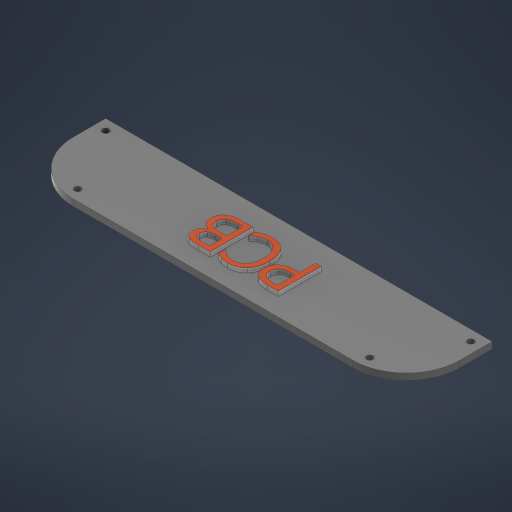
# Autodesk Inventor part: pcb
Saved by Autodesk Inventor 2024 (Build 280153000, 153)
## iProperties
Created: 2023-07-13
Part Number: pcb
Material: 일반
Document SubType Name: Modeling
Designer: 6gioc
Density: 1 g/cm^3
Appearance: 기본값
Author: 6gioc
Autodesk Inventor part; units mm, degrees
ref_plane "YZ Plane" through (0, 0, 0) normal (1, 0, 0) x (0, 1, 0)
ref_plane "XZ Plane" through (0, 0, 0) normal (0, 1, 0) x (-1, 0, 0)
ref_plane "XY Plane" through (0, 0, 0) normal (0, 0, 1) x (1, 0, 0)
sketch "스케치1" plane through (0, 0, 0) normal (0, 1, 0) x (-1, 0, 0)
  line L0 (-25, 0) -> (-155, 0)
  line L1 (-180, -25) -> (-180, -40)
  line L2 (-180, -40) -> (0, -40)
  line L3 (0, -40) -> (0, -25)
  arc A0 (0, -25) -> (-25, 0) centre (-25, -25) ccw
  arc A1 (-155, 0) -> (-180, -25) centre (-155, -25) ccw
  circle A2 centre (-5, -35) radius 1.5
  circle A3 centre (-5, -35) radius 2.5
  circle A4 centre (-5, -22) radius 1.5
  circle A5 centre (-5, -22) radius 2.5
  circle A6 centre (-22, -5) radius 1.5
  circle A7 centre (-22, -5) radius 2.5
  line L4 (-90, -40) -> (-90, 0)
  circle A8 centre (-90, -35) radius 2.5
  circle A9 centre (-90, -5) radius 2.5
  circle A10 centre (-47.5, -35) radius 2.5
  circle A11 centre (-175, -35) radius 1.5
  circle A12 centre (-175, -35) radius 2.5
  circle A13 centre (-175, -22) radius 1.5
  circle A14 centre (-175, -22) radius 2.5
  circle A15 centre (-158, -5) radius 1.5
  circle A16 centre (-158, -5) radius 2.5
  circle A17 centre (-132.5, -35) radius 2.5
  point P0 (0, 0)
  point P1 (-180, 0)
  dimension "d0" = 180
  dimension "d1" = 40
  dimension "d2" = 25
  dimension "d3" = 3
  dimension "d4" = 5
  dimension "d5" = 3
  dimension "d6" = 5
  dimension "d7" = 3
  dimension "d8" = 5
  dimension "d9" = 5
  dimension "d10" = 5
  dimension "d11" = 5
  dimension "d12" = 5
  dimension "d13" = 5
  dimension "d14" = 5
  dimension "d15" = 5
  dimension "d16" = 5
  dimension "d17" = 5
  dimension "d18" = 85
  dimension "d19" = 42.5
  dimension "d20" = 3
  dimension "d21" = 3
  constraints: 18 centre point, 10 end point, 7 symmetric about line, 6 coincident, 6 point on line, 4 point on circle, 4 tangent, 2 midpoint, 2 parallel, 1 equal radius, 1 horizontal, 1 horizontal alignment, 1 perpendicular, 7 other
  measures "d0" distance of L2.end L1.end
  measures "d1" distance of L1.end point (-180, 0)
  measures "d2" radius of A0
  measures "d3" diameter of A2
  measures "d4" diameter of A3
  measures "d5" diameter of A4
  measures "d6" diameter of A5
  measures "d7" diameter of A6
  measures "d8" diameter of A7
  measures "d9" diameter of A8
  measures "d10" diameter of A9
  measures "d11" diameter of A10
  measures "d12" distance from line of L2 A3.centre
  measures "d13" distance from line of A3.centre L3
  measures "d14" distance from line of L3 A5.centre
  measures "d15" distance from line of L0 A7.centre
  measures "d16" distance from line of L2 A8.centre
  measures "d17" distance from line of L0 A9.centre
  measures "d18" distance of A8.centre A2.centre
  measures "d19" distance of A8.centre A10.centre
  measures "d20" horizontal distance of L0.start A7.centre
  measures "d21" vertical distance of L3.end A5.centre
extrude "돌출1" add sketch "스케치1" along normal blind 3 contours A0 L3 L2 L4 A8 A9 L0 | L4 A9 A8 L2 L1 A1 L0 | A9 L4 | L4 A9 | A8 L4 | L4 A8 | A3 | A4 | A5 | A7 | A10 | A12 | A13 | A14 | A16 | A17
sketch "스케치2" plane through (0, 3, 0) normal (0, 1, 0) x (1, 0, 0)
  line L0 (113.9465, 8.0671) -> (66.0535, 8.0671) construction
  line L1 (66.0535, 8.0671) -> (66.0535, 31.9329) construction
  line L2 (66.0535, 31.9329) -> (113.9465, 31.9329) construction
  line L3 (113.9465, 31.9329) -> (113.9465, 8.0671) construction
  line L4 (0, 40) -> (0, 25) projected
  line L5 (180, 40) -> (0, 40) projected
  spline S0 degree 2 poles (99.2788, 14.4529) (99.2788, 15.7494) (100.2026, 18.0833) (101.0292, 18.8937) knots 0 0 0 1 2 2 2
  spline S1 degree 2 poles (101.0292, 18.8937) (102.0664, 19.9148) (104.8703, 20.9682) (107.0097, 20.9682) knots 0 0 0 1 2 2 2
  line L6 (107.0097, 20.9682) -> (109.2626, 20.9682)
  line L7 (109.2626, 20.9682) -> (109.2626, 28.4237)
  line L8 (109.2626, 28.4237) -> (111.9206, 28.4237)
  line L9 (111.9206, 28.4237) -> (111.9206, 8.4237)
  line L10 (111.9206, 8.4237) -> (106.8963, 8.4237)
  spline S2 degree 2 poles (106.8963, 8.4237) (105.1135, 8.4237) (102.6175, 9.0071) (101.6613, 9.6717) knots 0 0 0 1 2 2 2
  spline S3 degree 2 poles (101.6613, 9.6717) (100.5429, 10.4334) (99.2788, 12.7835) (99.2788, 14.4529) knots 0 0 0 1 2 2 2
  spline S4 degree 2 poles (102.0502, 14.5339) (102.0502, 13.4966) (102.7634, 11.9731) (103.4927, 11.4869) knots 0 0 0 1 2 2 2
  spline S5 degree 2 poles (103.4927, 11.4869) (104.1248, 11.0655) (105.8104, 10.7251) (107.0583, 10.7251) knots 0 0 0 1 2 2 2
  line L11 (107.0583, 10.7251) -> (109.2626, 10.7251)
  line L12 (109.2626, 10.7251) -> (109.2626, 18.6992)
  line L13 (109.2626, 18.6992) -> (107.4473, 18.6992)
  spline S6 degree 2 poles (107.4473, 18.6992) (105.8266, 18.6992) (103.8331, 18.1806) (103.1848, 17.4999) knots 0 0 0 1 2 2 2
  spline S7 degree 2 poles (103.1848, 17.4999) (102.5851, 16.9002) (102.0502, 15.4901) (102.0502, 14.5339) knots 0 0 0 1 2 2 2
  spline S8 degree 2 poles (88.9384, 28.7802) (90.8833, 28.7802) (94.1734, 27.4674) (95.3728, 26.1546) knots 0 0 0 1 2 2 2
  spline S9 degree 2 poles (95.3728, 26.1546) (96.5721, 24.858) (97.8849, 20.9682) (97.8849, 18.4399) knots 0 0 0 1 2 2 2
  spline S10 degree 2 poles (97.8849, 18.4399) (97.8849, 15.9277) (96.6045, 12.2) (95.389, 10.8224) knots 0 0 0 1 2 2 2
  spline S11 degree 2 poles (95.389, 10.8224) (94.1896, 9.4772) (90.9157, 8.0671) (88.8898, 8.0671) knots 0 0 0 1 2 2 2
  spline S12 degree 2 poles (88.8898, 8.0671) (87.8849, 8.0671) (86.1183, 8.3588) (85.3728, 8.5858) knots 0 0 0 1 2 2 2
  spline S13 degree 2 poles (85.3728, 8.5858) (84.7245, 8.7964) (83.3793, 9.3961) (82.7147, 9.7527) knots 0 0 0 1 2 2 2
  line L14 (82.7147, 9.7527) -> (82.7147, 12.9618)
  line L15 (82.7147, 12.9618) -> (82.9254, 12.9618)
  spline S14 degree 2 poles (82.9254, 12.9618) (83.282, 12.6376) (84.3841, 11.73) (85.1783, 11.2924) knots 0 0 0 1 2 2 2
  spline S15 degree 2 poles (85.1783, 11.2924) (85.94, 10.871) (87.7391, 10.3362) (88.906, 10.3362) knots 0 0 0 1 2 2 2
  spline S16 degree 2 poles (88.906, 10.3362) (90.1864, 10.3362) (92.4716, 11.3896) (93.3306, 12.3945) knots 0 0 0 1 2 2 2
  spline S17 degree 2 poles (93.3306, 12.3945) (94.1734, 13.4156) (95.1135, 16.5112) (95.1135, 18.4399) knots 0 0 0 1 2 2 2
  spline S18 degree 2 poles (95.1135, 18.4399) (95.1135, 20.4982) (94.1248, 23.4642) (93.2658, 24.4853) knots 0 0 0 1 2 2 2
  spline S19 degree 2 poles (93.2658, 24.4853) (92.423, 25.4739) (90.1702, 26.4788) (88.906, 26.4788) knots 0 0 0 1 2 2 2
  spline S20 degree 2 poles (88.906, 26.4788) (87.7553, 26.4788) (85.7942, 25.9115) (85.0324, 25.4901) knots 0 0 0 1 2 2 2
  spline S21 degree 2 poles (85.0324, 25.4901) (84.3031, 25.0687) (83.2172, 24.1935) (82.9092, 23.8856) knots 0 0 0 1 2 2 2
  line L16 (82.9092, 23.8856) -> (82.7147, 23.8856)
  line L17 (82.7147, 23.8856) -> (82.7147, 27.0623)
  spline S22 degree 2 poles (82.7147, 27.0623) (83.3793, 27.3702) (84.5462, 27.9375) (85.3728, 28.1968) knots 0 0 0 1 2 2 2
  spline S23 degree 2 poles (85.3728, 28.1968) (86.248, 28.4885) (87.7391, 28.7802) (88.9384, 28.7802) knots 0 0 0 1 2 2 2
  spline S24 degree 2 poles (66.6694, 22.2811) (66.6694, 23.7721) (67.8039, 26.0574) (68.7439, 26.8029) knots 0 0 0 1 2 2 2
  spline S25 degree 2 poles (68.7439, 26.8029) (69.8784, 27.6781) (72.4554, 28.4237) (74.4976, 28.4237) knots 0 0 0 1 2 2 2
  line L18 (74.4976, 28.4237) -> (80.235, 28.4237)
  line L19 (80.235, 28.4237) -> (80.235, 8.4237)
  line L20 (80.235, 8.4237) -> (74.9352, 8.4237)
  spline S26 degree 2 poles (74.9352, 8.4237) (72.7958, 8.4237) (70.6564, 8.6992) (69.684, 9.234) knots 0 0 0 1 2 2 2
  spline S27 degree 2 poles (69.684, 9.234) (68.5981, 9.8013) (67.6094, 11.6652) (67.6094, 12.9293) knots 0 0 0 1 2 2 2
  spline S28 degree 2 poles (67.6094, 12.9293) (67.6094, 14.3394) (69.1005, 16.576) (70.4133, 17.2081) knots 0 0 0 1 2 2 2
  line L21 (70.4133, 17.2081) -> (70.4133, 17.3054)
  spline S29 degree 2 poles (70.4133, 17.3054) (68.6305, 17.7916) (66.6694, 20.3686) (66.6694, 22.2811) knots 0 0 0 1 2 2 2
  spline S30 degree 2 poles (69.4408, 22.3945) (69.4408, 21.26) (70.0891, 19.8013) (71.0616, 19.2827) knots 0 0 0 1 2 2 2
  spline S31 degree 2 poles (71.0616, 19.2827) (71.6937, 18.9585) (73.1848, 18.764) (74.5624, 18.764) knots 0 0 0 1 2 2 2
  line L22 (74.5624, 18.764) -> (77.577, 18.764)
  line L23 (77.577, 18.764) -> (77.577, 26.1546)
  line L24 (77.577, 26.1546) -> (75.4214, 26.1546)
  spline S32 degree 2 poles (75.4214, 26.1546) (73.671, 26.1546) (71.6613, 25.8305) (70.8833, 25.3118) knots 0 0 0 1 2 2 2
  spline S33 degree 2 poles (70.8833, 25.3118) (70.1378, 24.777) (69.4408, 23.448) (69.4408, 22.3945) knots 0 0 0 1 2 2 2
  spline S34 degree 2 poles (70.3809, 13.3021) (70.3809, 12.589) (70.8671, 11.5193) (71.4019, 11.2114) knots 0 0 0 1 2 2 2
  spline S35 degree 2 poles (71.4019, 11.2114) (72.0502, 10.8548) (73.6224, 10.6927) (75.0324, 10.6927) knots 0 0 0 1 2 2 2
  line L25 (75.0324, 10.6927) -> (77.577, 10.6927)
  line L26 (77.577, 10.6927) -> (77.577, 16.5436)
  line L27 (77.577, 16.5436) -> (74.5624, 16.5436)
  spline S36 degree 2 poles (74.5624, 16.5436) (73.3144, 16.5436) (72.1313, 16.2843) (71.4992, 15.8791) knots 0 0 0 1 2 2 2
  spline S37 degree 2 poles (71.4992, 15.8791) (70.8833, 15.4901) (70.3809, 14.2422) (70.3809, 13.3021) knots 0 0 0 1 2 2 2
  point P0 (0, 0)
  point P1 (90, 8.0671)
  point P2 (66.0535, 20)
  dimension "d24" = 90
  dimension "d25" = 20
  constraints: 2 midpoint, 2 other
  measures "d24" distance from line of L4 point (90, 8.067)
  measures "d25" distance from line of L5 point (66.053, 20)
extrude "돌출2" add sketch "스케치2" along normal blind 2
